Autodesk Fusion 360 part; units mm, degrees
note: some values were not read from the file. Set by a fixed rule: which face or edge a step refers to.
(part 2 of 2)
  spline S256 degree 2 poles (23.5362, -10.063) (23.4772, -9.991) (23.4772, -9.8812) knots 0 0 0 1 1 1
  spline S257 degree 2 poles (23.4772, -9.8812) (23.4772, -9.7366) (23.5808, -9.6541) knots 0 0 0 1 1 1
  spline S258 degree 2 poles (23.5808, -9.6541) (23.7057, -9.5552) (23.9874, -9.5552) knots 0 0 0 1 1 1
  spline S259 degree 2 poles (23.9874, -9.6814) (23.7411, -9.6814) (23.6596, -9.739) knots 0 0 0 1 1 1
  spline S260 degree 2 poles (23.6596, -9.739) (23.5781, -9.7966) (23.5781, -9.8812) knots 0 0 0 1 1 1
  spline S261 degree 2 poles (23.5781, -9.8812) (23.5781, -9.9658) (23.66, -10.0234) knots 0 0 0 1 1 1
  spline S262 degree 2 poles (23.66, -10.0234) (23.7418, -10.0811) (23.9874, -10.0811) knots 0 0 0 1 1 1
  spline S263 degree 2 poles (23.9874, -10.0811) (24.2343, -10.0811) (24.3155, -10.0234) knots 0 0 0 1 1 1
  spline S264 degree 2 poles (24.3155, -10.0234) (24.3967, -9.9658) (24.3967, -9.8799) knots 0 0 0 1 1 1
  spline S265 degree 2 poles (24.3967, -9.8799) (24.3967, -9.7953) (24.325, -9.7448) knots 0 0 0 1 1 1
  spline S266 degree 2 poles (24.325, -9.7448) (24.2336, -9.6814) (23.9874, -9.6814) knots 0 0 0 1 1 1
  line L84 (23.4942, -14.607) -> (23.7336, -14.607)
  line L85 (23.7336, -14.607) -> (23.7336, -14.1732)
  line L86 (23.7336, -14.1732) -> (23.8462, -14.1732)
  line L87 (23.8462, -14.1732) -> (24.4942, -14.6295)
  line L88 (24.4942, -14.6295) -> (24.4942, -14.7298)
  line L89 (24.4942, -14.7298) -> (23.8462, -14.7298)
  line L90 (23.8462, -14.7298) -> (23.8462, -14.8648)
  line L91 (23.8462, -14.8648) -> (23.7336, -14.8648)
  line L92 (23.7336, -14.8648) -> (23.7336, -14.7298)
  line L93 (23.7336, -14.7298) -> (23.4942, -14.7298)
  line L94 (23.4942, -14.7298) -> (23.4942, -14.607)
  line L95 (23.8462, -14.607) -> (24.2971, -14.607)
  line L96 (24.2971, -14.607) -> (23.8462, -14.2939)
  line L97 (23.8462, -14.2939) -> (23.8462, -14.607)
  spline S267 degree 2 poles (23.9874, -14.9904) (24.1647, -14.9904) (24.2729, -15.0269) knots 0 0 0 1 1 1
  spline S268 degree 2 poles (24.2729, -15.0269) (24.381, -15.0633) (24.4396, -15.1353) knots 0 0 0 1 1 1
  spline S269 degree 2 poles (24.4396, -15.1353) (24.4983, -15.2073) (24.4983, -15.3164) knots 0 0 0 1 1 1
  spline S270 degree 2 poles (24.4983, -15.3164) (24.4983, -15.3969) (24.4659, -15.4576) knots 0 0 0 1 1 1
  spline S271 degree 2 poles (24.4659, -15.4576) (24.4335, -15.5183) (24.3724, -15.5579) knots 0 0 0 1 1 1
  spline S272 degree 2 poles (24.3724, -15.5579) (24.3114, -15.5975) (24.2237, -15.62) knots 0 0 0 1 1 1
  spline S273 degree 2 poles (24.2237, -15.62) (24.1361, -15.6425) (23.9874, -15.6425) knots 0 0 0 1 1 1
  spline S274 degree 2 poles (23.9874, -15.6425) (23.8114, -15.6425) (23.7033, -15.6063) knots 0 0 0 1 1 1
  spline S275 degree 2 poles (23.7033, -15.6063) (23.5952, -15.5702) (23.5362, -15.4982) knots 0 0 0 1 1 1
  spline S276 degree 2 poles (23.5362, -15.4982) (23.4772, -15.4262) (23.4772, -15.3164) knots 0 0 0 1 1 1
  spline S277 degree 2 poles (23.4772, -15.3164) (23.4772, -15.1718) (23.5808, -15.0893) knots 0 0 0 1 1 1
  spline S278 degree 2 poles (23.5808, -15.0893) (23.7057, -14.9904) (23.9874, -14.9904) knots 0 0 0 1 1 1
  spline S279 degree 2 poles (23.9874, -15.1166) (23.7411, -15.1166) (23.6596, -15.1742) knots 0 0 0 1 1 1
  spline S280 degree 2 poles (23.6596, -15.1742) (23.5781, -15.2318) (23.5781, -15.3164) knots 0 0 0 1 1 1
  spline S281 degree 2 poles (23.5781, -15.3164) (23.5781, -15.401) (23.66, -15.4586) knots 0 0 0 1 1 1
  spline S282 degree 2 poles (23.66, -15.4586) (23.7418, -15.5163) (23.9874, -15.5163) knots 0 0 0 1 1 1
  spline S283 degree 2 poles (23.9874, -15.5163) (24.2343, -15.5163) (24.3155, -15.4586) knots 0 0 0 1 1 1
  spline S284 degree 2 poles (24.3155, -15.4586) (24.3967, -15.401) (24.3967, -15.3151) knots 0 0 0 1 1 1
  spline S285 degree 2 poles (24.3967, -15.3151) (24.3967, -15.2305) (24.325, -15.18) knots 0 0 0 1 1 1
  spline S286 degree 2 poles (24.325, -15.18) (24.2336, -15.1166) (23.9874, -15.1166) knots 0 0 0 1 1 1
  spline S287 degree 2 poles (23.9874, -15.7673) (24.1647, -15.7673) (24.2729, -15.8038) knots 0 0 0 1 1 1
  spline S288 degree 2 poles (24.2729, -15.8038) (24.381, -15.8403) (24.4396, -15.9123) knots 0 0 0 1 1 1
  spline S289 degree 2 poles (24.4396, -15.9123) (24.4983, -15.9842) (24.4983, -16.0934) knots 0 0 0 1 1 1
  spline S290 degree 2 poles (24.4983, -16.0934) (24.4983, -16.1739) (24.4659, -16.2346) knots 0 0 0 1 1 1
  spline S291 degree 2 poles (24.4659, -16.2346) (24.4335, -16.2953) (24.3724, -16.3348) knots 0 0 0 1 1 1
  spline S292 degree 2 poles (24.3724, -16.3348) (24.3114, -16.3744) (24.2237, -16.3969) knots 0 0 0 1 1 1
  spline S293 degree 2 poles (24.2237, -16.3969) (24.1361, -16.4194) (23.9874, -16.4194) knots 0 0 0 1 1 1
  spline S294 degree 2 poles (23.9874, -16.4194) (23.8114, -16.4194) (23.7033, -16.3833) knots 0 0 0 1 1 1
  spline S295 degree 2 poles (23.7033, -16.3833) (23.5952, -16.3471) (23.5362, -16.2751) knots 0 0 0 1 1 1
  spline S296 degree 2 poles (23.5362, -16.2751) (23.4772, -16.2032) (23.4772, -16.0934) knots 0 0 0 1 1 1
  spline S297 degree 2 poles (23.4772, -16.0934) (23.4772, -15.9487) (23.5808, -15.8662) knots 0 0 0 1 1 1
  spline S298 degree 2 poles (23.5808, -15.8662) (23.7057, -15.7673) (23.9874, -15.7673) knots 0 0 0 1 1 1
  spline S299 degree 2 poles (23.9874, -15.8935) (23.7411, -15.8935) (23.6596, -15.9511) knots 0 0 0 1 1 1
  spline S300 degree 2 poles (23.6596, -15.9511) (23.5781, -16.0088) (23.5781, -16.0934) knots 0 0 0 1 1 1
  spline S301 degree 2 poles (23.5781, -16.0934) (23.5781, -16.1779) (23.66, -16.2356) knots 0 0 0 1 1 1
  spline S302 degree 2 poles (23.66, -16.2356) (23.7418, -16.2932) (23.9874, -16.2932) knots 0 0 0 1 1 1
  spline S303 degree 2 poles (23.9874, -16.2932) (24.2343, -16.2932) (24.3155, -16.2356) knots 0 0 0 1 1 1
  spline S304 degree 2 poles (24.3155, -16.2356) (24.3967, -16.1779) (24.3967, -16.092) knots 0 0 0 1 1 1
  spline S305 degree 2 poles (24.3967, -16.092) (24.3967, -16.0074) (24.325, -15.9569) knots 0 0 0 1 1 1
  spline S306 degree 2 poles (24.325, -15.9569) (24.2336, -15.8935) (23.9874, -15.8935) knots 0 0 0 1 1 1
  line L98 (18.9618, -23.4484) -> (18.9618, -24.4484)
  line L99 (18.9618, -24.4484) -> (18.5184, -24.4484)
  spline S307 degree 2 poles (18.5184, -24.4484) (18.3847, -24.4484) (18.3151, -24.4215) knots 0 0 0 1 1 1
  spline S308 degree 2 poles (18.3151, -24.4215) (18.2455, -24.3945) (18.2039, -24.3263) knots 0 0 0 1 1 1
  spline S309 degree 2 poles (18.2039, -24.3263) (18.1623, -24.2581) (18.1623, -24.1755) knots 0 0 0 1 1 1
  spline S310 degree 2 poles (18.1623, -24.1755) (18.1623, -24.0691) (18.2312, -23.9961) knots 0 0 0 1 1 1
  spline S311 degree 2 poles (18.2312, -23.9961) (18.3001, -23.9232) (18.444, -23.9034) knots 0 0 0 1 1 1
  spline S312 degree 2 poles (18.444, -23.9034) (18.3915, -23.8781) (18.3642, -23.8536) knots 0 0 0 1 1 1
  spline S313 degree 2 poles (18.3642, -23.8536) (18.3062, -23.8004) (18.2544, -23.7206) knots 0 0 0 1 1 1
  line L100 (18.2544, -23.7206) -> (18.0805, -23.4484)
  line L101 (18.0805, -23.4484) -> (18.2469, -23.4484)
  line L102 (18.2469, -23.4484) -> (18.3792, -23.6564)
  spline S314 degree 2 poles (18.3792, -23.6564) (18.4372, -23.7465) (18.4747, -23.7942) knots 0 0 0 1 1 1
  spline S315 degree 2 poles (18.4747, -23.7942) (18.5122, -23.842) (18.5419, -23.8611) knots 0 0 0 1 1 1
  spline S316 degree 2 poles (18.5419, -23.8611) (18.5716, -23.8802) (18.6023, -23.8877) knots 0 0 0 1 1 1
  spline S317 degree 2 poles (18.6023, -23.8877) (18.6248, -23.8925) (18.676, -23.8925) knots 0 0 0 1 1 1
  line L103 (18.676, -23.8925) -> (18.8294, -23.8925)
  line L104 (18.8294, -23.8925) -> (18.8294, -23.4484)
  line L105 (18.8294, -23.4484) -> (18.9618, -23.4484)
  line L106 (18.8294, -24.0071) -> (18.545, -24.0071)
  spline S318 degree 2 poles (18.545, -24.0071) (18.4543, -24.0071) (18.4031, -24.0258) knots 0 0 0 1 1 1
  spline S319 degree 2 poles (18.4031, -24.0258) (18.3519, -24.0446) (18.3253, -24.0858) knots 0 0 0 1 1 1
  spline S320 degree 2 poles (18.3253, -24.0858) (18.2987, -24.1271) (18.2987, -24.1755) knots 0 0 0 1 1 1
  spline S321 degree 2 poles (18.2987, -24.1755) (18.2987, -24.2465) (18.3502, -24.2922) knots 0 0 0 1 1 1
  spline S322 degree 2 poles (18.3502, -24.2922) (18.4017, -24.3379) (18.5129, -24.3379) knots 0 0 0 1 1 1
  line L107 (18.5129, -24.3379) -> (18.8294, -24.3379)
  line L108 (18.8294, -24.3379) -> (18.8294, -24.0071)
  line L109 (17.4747, -23.6817) -> (17.3479, -23.666)
  spline S323 degree 2 poles (17.3479, -23.666) (17.3779, -23.5548) (17.459, -23.4934) knots 0 0 0 1 1 1
  spline S324 degree 2 poles (17.459, -23.4934) (17.5402, -23.432) (17.6664, -23.432) knots 0 0 0 1 1 1
  spline S325 degree 2 poles (17.6664, -23.432) (17.8253, -23.432) (17.9185, -23.5299) knots 0 0 0 1 1 1
  spline S326 degree 2 poles (17.9185, -23.5299) (18.0116, -23.6278) (18.0116, -23.8045) knots 0 0 0 1 1 1
  spline S327 degree 2 poles (18.0116, -23.8045) (18.0116, -23.9873) (17.9174, -24.0882) knots 0 0 0 1 1 1
  spline S328 degree 2 poles (17.9174, -24.0882) (17.8233, -24.1892) (17.6732, -24.1892) knots 0 0 0 1 1 1
  spline S329 degree 2 poles (17.6732, -24.1892) (17.5279, -24.1892) (17.4358, -24.0903) knots 0 0 0 1 1 1
  spline S330 degree 2 poles (17.4358, -24.0903) (17.3438, -23.9914) (17.3438, -23.812) knots 0 0 0 1 1 1
  spline S331 degree 2 poles (17.3438, -23.812) (17.3438, -23.8011) (17.3444, -23.7792) knots 0 0 0 1 1 1
  line L110 (17.3444, -23.7792) -> (17.8847, -23.7792)
  spline S332 degree 2 poles (17.8847, -23.7792) (17.8779, -23.6599) (17.8172, -23.5964) knots 0 0 0 1 1 1
  spline S333 degree 2 poles (17.8172, -23.5964) (17.7564, -23.533) (17.6657, -23.533) knots 0 0 0 1 1 1
  spline S334 degree 2 poles (17.6657, -23.533) (17.5982, -23.533) (17.5504, -23.5685) knots 0 0 0 1 1 1
  spline S335 degree 2 poles (17.5504, -23.5685) (17.5027, -23.6039) (17.4747, -23.6817) knots 0 0 0 1 1 1
  line L111 (17.8779, -23.8802) -> (17.4734, -23.8802)
  spline S336 degree 2 poles (17.4734, -23.8802) (17.4815, -23.9716) (17.5197, -24.0173) knots 0 0 0 1 1 1
  spline S337 degree 2 poles (17.5197, -24.0173) (17.5784, -24.0882) (17.6719, -24.0882) knots 0 0 0 1 1 1
  spline S338 degree 2 poles (17.6719, -24.0882) (17.7564, -24.0882) (17.8141, -24.0316) knots 0 0 0 1 1 1
  spline S339 degree 2 poles (17.8141, -24.0316) (17.8717, -23.975) (17.8779, -23.8802) knots 0 0 0 1 1 1
  line L112 (17.2428, -23.6646) -> (17.1214, -23.6837)
  spline S340 degree 2 poles (17.1214, -23.6837) (17.1112, -23.6107) (17.0644, -23.5719) knots 0 0 0 1 1 1
  spline S341 degree 2 poles (17.0644, -23.5719) (17.0177, -23.533) (16.9338, -23.533) knots 0 0 0 1 1 1
  spline S342 degree 2 poles (16.9338, -23.533) (16.8492, -23.533) (16.8083, -23.5674) knots 0 0 0 1 1 1
  spline S343 degree 2 poles (16.8083, -23.5674) (16.7674, -23.6019) (16.7674, -23.6483) knots 0 0 0 1 1 1
  spline S344 degree 2 poles (16.7674, -23.6483) (16.7674, -23.6899) (16.8035, -23.7137) knots 0 0 0 1 1 1
  spline S345 degree 2 poles (16.8035, -23.7137) (16.8288, -23.7301) (16.929, -23.7554) knots 0 0 0 1 1 1
  spline S346 degree 2 poles (16.929, -23.7554) (17.0641, -23.7895) (17.1163, -23.8144) knots 0 0 0 1 1 1
  spline S347 degree 2 poles (17.1163, -23.8144) (17.1685, -23.8393) (17.1954, -23.8833) knots 0 0 0 1 1 1
  spline S348 degree 2 poles (17.1954, -23.8833) (17.2223, -23.9273) (17.2223, -23.9805) knots 0 0 0 1 1 1
  spline S349 degree 2 poles (17.2223, -23.9805) (17.2223, -24.0289) (17.2002, -24.0702) knots 0 0 0 1 1 1
  spline S350 degree 2 poles (17.2002, -24.0702) (17.178, -24.1114) (17.1398, -24.1387) knots 0 0 0 1 1 1
  spline S351 degree 2 poles (17.1398, -24.1387) (17.1112, -24.1599) (17.0617, -24.1745) knots 0 0 0 1 1 1
  spline S352 degree 2 poles (17.0617, -24.1745) (17.0122, -24.1892) (16.9556, -24.1892) knots 0 0 0 1 1 1
  spline S353 degree 2 poles (16.9556, -24.1892) (16.8704, -24.1892) (16.8059, -24.1646) knots 0 0 0 1 1 1
  spline S354 degree 2 poles (16.8059, -24.1646) (16.7414, -24.1401) (16.7107, -24.0981) knots 0 0 0 1 1 1
  spline S355 degree 2 poles (16.7107, -24.0981) (16.68, -24.0562) (16.6685, -23.9859) knots 0 0 0 1 1 1
  line L113 (16.6685, -23.9859) -> (16.7885, -23.9695)
  spline S356 degree 2 poles (16.7885, -23.9695) (16.7967, -24.0255) (16.8359, -24.0569) knots 0 0 0 1 1 1
  spline S357 degree 2 poles (16.8359, -24.0569) (16.8751, -24.0882) (16.9468, -24.0882) knots 0 0 0 1 1 1
  spline S358 degree 2 poles (16.9468, -24.0882) (17.0313, -24.0882) (17.0675, -24.0603) knots 0 0 0 1 1 1
  spline S359 degree 2 poles (17.0675, -24.0603) (17.1037, -24.0323) (17.1037, -23.9948) knots 0 0 0 1 1 1
  spline S360 degree 2 poles (17.1037, -23.9948) (17.1037, -23.9709) (17.0886, -23.9518) knots 0 0 0 1 1 1
  spline S361 degree 2 poles (17.0886, -23.9518) (17.0736, -23.932) (17.0416, -23.9191) knots 0 0 0 1 1 1
  spline S362 degree 2 poles (17.0416, -23.9191) (17.0232, -23.9122) (16.9331, -23.8877) knots 0 0 0 1 1 1
  spline S363 degree 2 poles (16.9331, -23.8877) (16.8028, -23.8529) (16.7513, -23.8307) knots 0 0 0 1 1 1
  spline S364 degree 2 poles (16.7513, -23.8307) (16.6998, -23.8086) (16.6705, -23.7663) knots 0 0 0 1 1 1
  spline S365 degree 2 poles (16.6705, -23.7663) (16.6412, -23.724) (16.6412, -23.6612) knots 0 0 0 1 1 1
  spline S366 degree 2 poles (16.6412, -23.6612) (16.6412, -23.5998) (16.677, -23.5456) knots 0 0 0 1 1 1
  spline S367 degree 2 poles (16.677, -23.5456) (16.7128, -23.4914) (16.7803, -23.4617) knots 0 0 0 1 1 1
  spline S368 degree 2 poles (16.7803, -23.4617) (16.8479, -23.432) (16.9331, -23.432) knots 0 0 0 1 1 1
  spline S369 degree 2 poles (16.9331, -23.432) (17.0743, -23.432) (17.1483, -23.4907) knots 0 0 0 1 1 1
  spline S370 degree 2 poles (17.1483, -23.4907) (17.2223, -23.5494) (17.2428, -23.6646) knots 0 0 0 1 1 1
  spline S371 degree 2 poles (16.5409, -23.8106) (16.5409, -24.0118) (16.429, -24.1087) knots 0 0 0 1 1 1
  spline S372 degree 2 poles (16.429, -24.1087) (16.3356, -24.1892) (16.2012, -24.1892) knots 0 0 0 1 1 1
  spline S373 degree 2 poles (16.2012, -24.1892) (16.0518, -24.1892) (15.957, -24.0913) knots 0 0 0 1 1 1
  spline S374 degree 2 poles (15.957, -24.0913) (15.8622, -23.9934) (15.8622, -23.8208) knots 0 0 0 1 1 1
  spline S375 degree 2 poles (15.8622, -23.8208) (15.8622, -23.681) (15.9041, -23.6009) knots 0 0 0 1 1 1
  spline S376 degree 2 poles (15.9041, -23.6009) (15.9461, -23.5207) (16.0262, -23.4764) knots 0 0 0 1 1 1
  spline S377 degree 2 poles (16.0262, -23.4764) (16.1064, -23.432) (16.2012, -23.432) knots 0 0 0 1 1 1
  spline S378 degree 2 poles (16.2012, -23.432) (16.3533, -23.432) (16.4471, -23.5296) knots 0 0 0 1 1 1
  spline S379 degree 2 poles (16.4471, -23.5296) (16.5409, -23.6271) (16.5409, -23.8106) knots 0 0 0 1 1 1
  spline S380 degree 2 poles (16.4147, -23.8106) (16.4147, -23.6715) (16.354, -23.6022) knots 0 0 0 1 1 1
  spline S381 degree 2 poles (16.354, -23.6022) (16.2933, -23.533) (16.2012, -23.533) knots 0 0 0 1 1 1
  spline S382 degree 2 poles (16.2012, -23.533) (16.1098, -23.533) (16.0491, -23.6026) knots 0 0 0 1 1 1
  spline S383 degree 2 poles (16.0491, -23.6026) (15.9884, -23.6721) (15.9884, -23.8147) knots 0 0 0 1 1 1
  spline S384 degree 2 poles (15.9884, -23.8147) (15.9884, -23.9491) (16.0494, -24.0183) knots 0 0 0 1 1 1
  spline S385 degree 2 poles (16.0494, -24.0183) (16.1105, -24.0876) (16.2012, -24.0876) knots 0 0 0 1 1 1
  spline S386 degree 2 poles (16.2012, -24.0876) (16.2933, -24.0876) (16.354, -24.0187) knots 0 0 0 1 1 1
  spline S387 degree 2 poles (16.354, -24.0187) (16.4147, -23.9498) (16.4147, -23.8106) knots 0 0 0 1 1 1
  line L114 (15.721, -23.4484) -> (15.721, -24.4484)
  line L115 (15.721, -24.4484) -> (15.5982, -24.4484)
  line L116 (15.5982, -24.4484) -> (15.5982, -23.4484)
  line L117 (15.5982, -23.4484) -> (15.721, -23.4484)
  line L118 (14.9331, -23.4484) -> (14.9331, -23.5548)
  spline S388 degree 2 poles (14.9331, -23.5548) (15.0177, -23.432) (15.163, -23.432) knots 0 0 0 1 1 1
  spline S389 degree 2 poles (15.163, -23.432) (15.2271, -23.432) (15.2827, -23.4566) knots 0 0 0 1 1 1
  spline S390 degree 2 poles (15.2827, -23.4566) (15.3383, -23.4811) (15.3652, -23.5183) knots 0 0 0 1 1 1
  spline S391 degree 2 poles (15.3652, -23.5183) (15.3922, -23.5555) (15.4031, -23.6094) knots 0 0 0 1 1 1
  spline S392 degree 2 poles (15.4031, -23.6094) (15.4106, -23.6455) (15.4106, -23.724) knots 0 0 0 1 1 1
  line L119 (15.4106, -23.724) -> (15.4106, -24.1728)
  line L120 (15.4106, -24.1728) -> (15.2878, -24.1728)
  line L121 (15.2878, -24.1728) -> (15.2878, -23.771)
  spline S393 degree 2 poles (15.2878, -23.771) (15.2878, -23.6749) (15.2803, -23.6414) knots 0 0 0 1 1 1
  spline S394 degree 2 poles (15.2803, -23.6414) (15.2687, -23.593) (15.2312, -23.5654) knots 0 0 0 1 1 1
  spline S395 degree 2 poles (15.2312, -23.5654) (15.1937, -23.5378) (15.1384, -23.5378) knots 0 0 0 1 1 1
  spline S396 degree 2 poles (15.1384, -23.5378) (15.0832, -23.5378) (15.0348, -23.5661) knots 0 0 0 1 1 1
  spline S397 degree 2 poles (15.0348, -23.5661) (14.9863, -23.5944) (14.9662, -23.6431) knots 0 0 0 1 1 1
  spline S398 degree 2 poles (14.9662, -23.6431) (14.9461, -23.6919) (14.9461, -23.7847) knots 0 0 0 1 1 1
  line L122 (14.9461, -23.7847) -> (14.9461, -24.1728)
  line L123 (14.9461, -24.1728) -> (14.8233, -24.1728)
  line L124 (14.8233, -24.1728) -> (14.8233, -23.4484)
  line L125 (14.8233, -23.4484) -> (14.9331, -23.4484)
  line L126 (14.3629, -23.5582) -> (14.3451, -23.4498)
  spline S399 degree 2 poles (14.3451, -23.4498) (14.397, -23.4388) (14.4379, -23.4388) knots 0 0 0 1 1 1
  spline S400 degree 2 poles (14.4379, -23.4388) (14.5047, -23.4388) (14.5416, -23.46) knots 0 0 0 1 1 1
  spline S401 degree 2 poles (14.5416, -23.46) (14.5784, -23.4811) (14.5934, -23.5156) knots 0 0 0 1 1 1
  spline S402 degree 2 poles (14.5934, -23.5156) (14.6084, -23.55) (14.6084, -23.6605) knots 0 0 0 1 1 1
  line L127 (14.6084, -23.6605) -> (14.6084, -24.0773)
  line L128 (14.6084, -24.0773) -> (14.6985, -24.0773)
  line L129 (14.6985, -24.0773) -> (14.6985, -24.1728)
  line L130 (14.6985, -24.1728) -> (14.6084, -24.1728)
  line L131 (14.6084, -24.1728) -> (14.6084, -24.3522)
  line L132 (14.6084, -24.3522) -> (14.4863, -24.4259)
  line L133 (14.4863, -24.4259) -> (14.4863, -24.1728)
  line L134 (14.4863, -24.1728) -> (14.3629, -24.1728)
  line L135 (14.3629, -24.1728) -> (14.3629, -24.0773)
  line L136 (14.3629, -24.0773) -> (14.4863, -24.0773)
  line L137 (14.4863, -24.0773) -> (14.4863, -23.6537)
  spline S403 degree 2 poles (14.4863, -23.6537) (14.4863, -23.6012) (14.4798, -23.5862) knots 0 0 0 1 1 1
  spline S404 degree 2 poles (14.4798, -23.5862) (14.4734, -23.5712) (14.4587, -23.5623) knots 0 0 0 1 1 1
  spline S405 degree 2 poles (14.4587, -23.5623) (14.444, -23.5534) (14.4167, -23.5534) knots 0 0 0 1 1 1
  spline S406 degree 2 poles (14.4167, -23.5534) (14.3963, -23.5534) (14.3629, -23.5582) knots 0 0 0 1 1 1
  line L138 (14.2421, -24.3072) -> (14.2421, -24.4484)
  line L139 (14.2421, -24.4484) -> (14.1193, -24.4484)
  line L140 (14.1193, -24.4484) -> (14.1193, -24.3072)
  line L141 (14.1193, -24.3072) -> (14.2421, -24.3072)
  line L142 (14.2421, -23.4484) -> (14.2421, -24.1728)
  line L143 (14.2421, -24.1728) -> (14.1193, -24.1728)
  line L144 (14.1193, -24.1728) -> (14.1193, -23.4484)
  line L145 (14.1193, -23.4484) -> (14.2421, -23.4484)
  spline S407 degree 2 poles (13.9781, -23.8106) (13.9781, -24.0118) (13.8663, -24.1087) knots 0 0 0 1 1 1
  spline S408 degree 2 poles (13.8663, -24.1087) (13.7728, -24.1892) (13.6384, -24.1892) knots 0 0 0 1 1 1
  spline S409 degree 2 poles (13.6384, -24.1892) (13.4891, -24.1892) (13.3942, -24.0913) knots 0 0 0 1 1 1
  spline S410 degree 2 poles (13.3942, -24.0913) (13.2994, -23.9934) (13.2994, -23.8208) knots 0 0 0 1 1 1
  spline S411 degree 2 poles (13.2994, -23.8208) (13.2994, -23.681) (13.3414, -23.6009) knots 0 0 0 1 1 1
  spline S412 degree 2 poles (13.3414, -23.6009) (13.3833, -23.5207) (13.4635, -23.4764) knots 0 0 0 1 1 1
  spline S413 degree 2 poles (13.4635, -23.4764) (13.5436, -23.432) (13.6384, -23.432) knots 0 0 0 1 1 1
  spline S414 degree 2 poles (13.6384, -23.432) (13.7906, -23.432) (13.8843, -23.5296) knots 0 0 0 1 1 1
  spline S415 degree 2 poles (13.8843, -23.5296) (13.9781, -23.6271) (13.9781, -23.8106) knots 0 0 0 1 1 1
  spline S416 degree 2 poles (13.8519, -23.8106) (13.8519, -23.6715) (13.7912, -23.6022) knots 0 0 0 1 1 1
  spline S417 degree 2 poles (13.7912, -23.6022) (13.7305, -23.533) (13.6384, -23.533) knots 0 0 0 1 1 1
  spline S418 degree 2 poles (13.6384, -23.533) (13.547, -23.533) (13.4863, -23.6026) knots 0 0 0 1 1 1
  spline S419 degree 2 poles (13.4863, -23.6026) (13.4256, -23.6721) (13.4256, -23.8147) knots 0 0 0 1 1 1
  spline S420 degree 2 poles (13.4256, -23.8147) (13.4256, -23.9491) (13.4867, -24.0183) knots 0 0 0 1 1 1
  spline S421 degree 2 poles (13.4867, -24.0183) (13.5477, -24.0876) (13.6384, -24.0876) knots 0 0 0 1 1 1
  spline S422 degree 2 poles (13.6384, -24.0876) (13.7305, -24.0876) (13.7912, -24.0187) knots 0 0 0 1 1 1
  spline S423 degree 2 poles (13.7912, -24.0187) (13.8519, -23.9498) (13.8519, -23.8106) knots 0 0 0 1 1 1
  line L146 (13.1555, -23.4484) -> (13.1555, -24.1728)
  line L147 (13.1555, -24.1728) -> (13.045, -24.1728)
  line L148 (13.045, -24.1728) -> (13.045, -24.0698)
  spline S424 degree 2 poles (13.045, -24.0698) (12.9652, -24.1892) (12.8144, -24.1892) knots 0 0 0 1 1 1
  spline S425 degree 2 poles (12.8144, -24.1892) (12.7489, -24.1892) (12.694, -24.1657) knots 0 0 0 1 1 1
  spline S426 degree 2 poles (12.694, -24.1657) (12.6391, -24.1421) (12.6118, -24.1039) knots 0 0 0 1 1 1
  spline S427 degree 2 poles (12.6118, -24.1039) (12.5846, -24.0657) (12.5736, -24.0132) knots 0 0 0 1 1 1
  spline S428 degree 2 poles (12.5736, -24.0132) (12.5668, -23.9791) (12.5668, -23.8938) knots 0 0 0 1 1 1
  line L149 (12.5668, -23.8938) -> (12.5668, -23.4484)
  line L150 (12.5668, -23.4484) -> (12.6896, -23.4484)
  line L151 (12.6896, -23.4484) -> (12.6896, -23.8891)
  spline S429 degree 2 poles (12.6896, -23.8891) (12.6896, -23.9641) (12.7039, -24.0013) knots 0 0 0 1 1 1
  spline S430 degree 2 poles (12.7039, -24.0013) (12.7182, -24.0384) (12.7547, -24.0606) knots 0 0 0 1 1 1
  spline S431 degree 2 poles (12.7547, -24.0606) (12.7912, -24.0828) (12.8403, -24.0828) knots 0 0 0 1 1 1
  spline S432 degree 2 poles (12.8403, -24.0828) (12.9188, -24.0828) (12.9758, -24.033) knots 0 0 0 1 1 1
  spline S433 degree 2 poles (12.9758, -24.033) (13.0327, -23.9832) (13.0327, -23.844) knots 0 0 0 1 1 1
  line L152 (13.0327, -23.844) -> (13.0327, -23.4484)
  line L153 (13.0327, -23.4484) -> (13.1555, -23.4484)
  line L154 (11.7223, -23.5582) -> (11.7046, -23.4498)
  spline S434 degree 2 poles (11.7046, -23.4498) (11.7564, -23.4388) (11.7974, -23.4388) knots 0 0 0 1 1 1
  spline S435 degree 2 poles (11.7974, -23.4388) (11.8642, -23.4388) (11.9011, -23.46) knots 0 0 0 1 1 1
  spline S436 degree 2 poles (11.9011, -23.46) (11.9379, -23.4811) (11.9529, -23.5156) knots 0 0 0 1 1 1
  spline S437 degree 2 poles (11.9529, -23.5156) (11.9679, -23.55) (11.9679, -23.6605) knots 0 0 0 1 1 1
  line L155 (11.9679, -23.6605) -> (11.9679, -24.0773)
  line L156 (11.9679, -24.0773) -> (12.0579, -24.0773)
  line L157 (12.0579, -24.0773) -> (12.0579, -24.1728)
  line L158 (12.0579, -24.1728) -> (11.9679, -24.1728)
  line L159 (11.9679, -24.1728) -> (11.9679, -24.3522)
  line L160 (11.9679, -24.3522) -> (11.8458, -24.4259)
  line L161 (11.8458, -24.4259) -> (11.8458, -24.1728)
  line L162 (11.8458, -24.1728) -> (11.7223, -24.1728)
  line L163 (11.7223, -24.1728) -> (11.7223, -24.0773)
  line L164 (11.7223, -24.0773) -> (11.8458, -24.0773)
  line L165 (11.8458, -24.0773) -> (11.8458, -23.6537)
  spline S438 degree 2 poles (11.8458, -23.6537) (11.8458, -23.6012) (11.8393, -23.5862) knots 0 0 0 1 1 1
  spline S439 degree 2 poles (11.8393, -23.5862) (11.8328, -23.5712) (11.8182, -23.5623) knots 0 0 0 1 1 1
  spline S440 degree 2 poles (11.8182, -23.5623) (11.8035, -23.5534) (11.7762, -23.5534) knots 0 0 0 1 1 1
  spline S441 degree 2 poles (11.7762, -23.5534) (11.7558, -23.5534) (11.7223, -23.5582) knots 0 0 0 1 1 1
  line L166 (11.1064, -23.6817) -> (10.9795, -23.666)
  spline S442 degree 2 poles (10.9795, -23.666) (11.0095, -23.5548) (11.0907, -23.4934) knots 0 0 0 1 1 1
  spline S443 degree 2 poles (11.0907, -23.4934) (11.1719, -23.432) (11.2981, -23.432) knots 0 0 0 1 1 1
  spline S444 degree 2 poles (11.2981, -23.432) (11.457, -23.432) (11.5501, -23.5299) knots 0 0 0 1 1 1
  spline S445 degree 2 poles (11.5501, -23.5299) (11.6432, -23.6278) (11.6432, -23.8045) knots 0 0 0 1 1 1
  spline S446 degree 2 poles (11.6432, -23.8045) (11.6432, -23.9873) (11.5491, -24.0882) knots 0 0 0 1 1 1
  spline S447 degree 2 poles (11.5491, -24.0882) (11.4549, -24.1892) (11.3049, -24.1892) knots 0 0 0 1 1 1
  spline S448 degree 2 poles (11.3049, -24.1892) (11.1596, -24.1892) (11.0675, -24.0903) knots 0 0 0 1 1 1
  spline S449 degree 2 poles (11.0675, -24.0903) (10.9754, -23.9914) (10.9754, -23.812) knots 0 0 0 1 1 1
  spline S450 degree 2 poles (10.9754, -23.812) (10.9754, -23.8011) (10.9761, -23.7792) knots 0 0 0 1 1 1
  line L167 (10.9761, -23.7792) -> (11.5163, -23.7792)
  spline S451 degree 2 poles (11.5163, -23.7792) (11.5095, -23.6599) (11.4488, -23.5964) knots 0 0 0 1 1 1
  spline S452 degree 2 poles (11.4488, -23.5964) (11.3881, -23.533) (11.2974, -23.533) knots 0 0 0 1 1 1
  spline S453 degree 2 poles (11.2974, -23.533) (11.2298, -23.533) (11.1821, -23.5685) knots 0 0 0 1 1 1
  spline S454 degree 2 poles (11.1821, -23.5685) (11.1343, -23.6039) (11.1064, -23.6817) knots 0 0 0 1 1 1
  line L168 (11.5095, -23.8802) -> (11.105, -23.8802)
  spline S455 degree 2 poles (11.105, -23.8802) (11.1132, -23.9716) (11.1514, -24.0173) knots 0 0 0 1 1 1
  spline S456 degree 2 poles (11.1514, -24.0173) (11.2101, -24.0882) (11.3035, -24.0882) knots 0 0 0 1 1 1
  spline S457 degree 2 poles (11.3035, -24.0882) (11.3881, -24.0882) (11.4457, -24.0316) knots 0 0 0 1 1 1
  spline S458 degree 2 poles (11.4457, -24.0316) (11.5034, -23.975) (11.5095, -23.8802) knots 0 0 0 1 1 1
  line L169 (10.8745, -23.6646) -> (10.753, -23.6837)
  spline S459 degree 2 poles (10.753, -23.6837) (10.7428, -23.6107) (10.6961, -23.5719) knots 0 0 0 1 1 1
  spline S460 degree 2 poles (10.6961, -23.5719) (10.6494, -23.533) (10.5655, -23.533) knots 0 0 0 1 1 1
  spline S461 degree 2 poles (10.5655, -23.533) (10.4809, -23.533) (10.4399, -23.5674) knots 0 0 0 1 1 1
  spline S462 degree 2 poles (10.4399, -23.5674) (10.399, -23.6019) (10.399, -23.6483) knots 0 0 0 1 1 1
  spline S463 degree 2 poles (10.399, -23.6483) (10.399, -23.6899) (10.4352, -23.7137) knots 0 0 0 1 1 1
  spline S464 degree 2 poles (10.4352, -23.7137) (10.4604, -23.7301) (10.5607, -23.7554) knots 0 0 0 1 1 1
  spline S465 degree 2 poles (10.5607, -23.7554) (10.6957, -23.7895) (10.7479, -23.8144) knots 0 0 0 1 1 1
  spline S466 degree 2 poles (10.7479, -23.8144) (10.8001, -23.8393) (10.827, -23.8833) knots 0 0 0 1 1 1
  spline S467 degree 2 poles (10.827, -23.8833) (10.854, -23.9273) (10.854, -23.9805) knots 0 0 0 1 1 1
  spline S468 degree 2 poles (10.854, -23.9805) (10.854, -24.0289) (10.8318, -24.0702) knots 0 0 0 1 1 1
  spline S469 degree 2 poles (10.8318, -24.0702) (10.8097, -24.1114) (10.7715, -24.1387) knots 0 0 0 1 1 1
  spline S470 degree 2 poles (10.7715, -24.1387) (10.7428, -24.1599) (10.6933, -24.1745) knots 0 0 0 1 1 1
  spline S471 degree 2 poles (10.6933, -24.1745) (10.6439, -24.1892) (10.5873, -24.1892) knots 0 0 0 1 1 1
  spline S472 degree 2 poles (10.5873, -24.1892) (10.502, -24.1892) (10.4376, -24.1646) knots 0 0 0 1 1 1
  spline S473 degree 2 poles (10.4376, -24.1646) (10.3731, -24.1401) (10.3424, -24.0981) knots 0 0 0 1 1 1
  spline S474 degree 2 poles (10.3424, -24.0981) (10.3117, -24.0562) (10.3001, -23.9859) knots 0 0 0 1 1 1
  line L170 (10.3001, -23.9859) -> (10.4202, -23.9695)
  spline S475 degree 2 poles (10.4202, -23.9695) (10.4283, -24.0255) (10.4676, -24.0569) knots 0 0 0 1 1 1
  spline S476 degree 2 poles (10.4676, -24.0569) (10.5068, -24.0882) (10.5784, -24.0882) knots 0 0 0 1 1 1
  spline S477 degree 2 poles (10.5784, -24.0882) (10.663, -24.0882) (10.6991, -24.0603) knots 0 0 0 1 1 1
  spline S478 degree 2 poles (10.6991, -24.0603) (10.7353, -24.0323) (10.7353, -23.9948) knots 0 0 0 1 1 1
  spline S479 degree 2 poles (10.7353, -23.9948) (10.7353, -23.9709) (10.7203, -23.9518) knots 0 0 0 1 1 1
  spline S480 degree 2 poles (10.7203, -23.9518) (10.7053, -23.932) (10.6732, -23.9191) knots 0 0 0 1 1 1
  spline S481 degree 2 poles (10.6732, -23.9191) (10.6548, -23.9122) (10.5648, -23.8877) knots 0 0 0 1 1 1
  spline S482 degree 2 poles (10.5648, -23.8877) (10.4345, -23.8529) (10.383, -23.8307) knots 0 0 0 1 1 1
  spline S483 degree 2 poles (10.383, -23.8307) (10.3315, -23.8086) (10.3021, -23.7663) knots 0 0 0 1 1 1
  spline S484 degree 2 poles (10.3021, -23.7663) (10.2728, -23.724) (10.2728, -23.6612) knots 0 0 0 1 1 1
  spline S485 degree 2 poles (10.2728, -23.6612) (10.2728, -23.5998) (10.3086, -23.5456) knots 0 0 0 1 1 1
  spline S486 degree 2 poles (10.3086, -23.5456) (10.3444, -23.4914) (10.412, -23.4617) knots 0 0 0 1 1 1
  spline S487 degree 2 poles (10.412, -23.4617) (10.4795, -23.432) (10.5648, -23.432) knots 0 0 0 1 1 1
  spline S488 degree 2 poles (10.5648, -23.432) (10.706, -23.432) (10.78, -23.4907) knots 0 0 0 1 1 1
  spline S489 degree 2 poles (10.78, -23.4907) (10.854, -23.5494) (10.8745, -23.6646) knots 0 0 0 1 1 1
  line L171 (9.8588, -23.5582) -> (9.841, -23.4498)
  spline S490 degree 2 poles (9.841, -23.4498) (9.8929, -23.4388) (9.9338, -23.4388) knots 0 0 0 1 1 1
  spline S491 degree 2 poles (9.9338, -23.4388) (10.0006, -23.4388) (10.0375, -23.46) knots 0 0 0 1 1 1
  spline S492 degree 2 poles (10.0375, -23.46) (10.0743, -23.4811) (10.0893, -23.5156) knots 0 0 0 1 1 1
  spline S493 degree 2 poles (10.0893, -23.5156) (10.1043, -23.55) (10.1043, -23.6605) knots 0 0 0 1 1 1
  line L172 (10.1043, -23.6605) -> (10.1043, -24.0773)
  line L173 (10.1043, -24.0773) -> (10.1944, -24.0773)
  line L174 (10.1944, -24.0773) -> (10.1944, -24.1728)
  line L175 (10.1944, -24.1728) -> (10.1043, -24.1728)
  line L176 (10.1043, -24.1728) -> (10.1043, -24.3522)
  line L177 (10.1043, -24.3522) -> (9.9822, -24.4259)
  line L178 (9.9822, -24.4259) -> (9.9822, -24.1728)
  line L179 (9.9822, -24.1728) -> (9.8588, -24.1728)
  line L180 (9.8588, -24.1728) -> (9.8588, -24.0773)
  line L181 (9.8588, -24.0773) -> (9.9822, -24.0773)
  line L182 (9.9822, -24.0773) -> (9.9822, -23.6537)
  spline S494 degree 2 poles (9.9822, -23.6537) (9.9822, -23.6012) (9.9758, -23.5862) knots 0 0 0 1 1 1
  spline S495 degree 2 poles (9.9758, -23.5862) (9.9693, -23.5712) (9.9546, -23.5623) knots 0 0 0 1 1 1
  spline S496 degree 2 poles (9.9546, -23.5623) (9.9399, -23.5534) (9.9127, -23.5534) knots 0 0 0 1 1 1
  spline S497 degree 2 poles (9.9127, -23.5534) (9.8922, -23.5534) (9.8588, -23.5582) knots 0 0 0 1 1 1
  spline S498 degree 2 poles (9.3847, -23.9416) (9.3847, -24.1189) (9.3482, -24.227) knots 0 0 0 1 1 1
  spline S499 degree 2 poles (9.3482, -24.227) (9.3117, -24.3352) (9.2397, -24.3938) knots 0 0 0 1 1 1
  spline S500 degree 2 poles (9.2397, -24.3938) (9.1678, -24.4525) (9.0586, -24.4525) knots 0 0 0 1 1 1
  spline S501 degree 2 poles (9.0586, -24.4525) (8.9781, -24.4525) (8.9174, -24.4201) knots 0 0 0 1 1 1
  spline S502 degree 2 poles (8.9174, -24.4201) (8.8567, -24.3877) (8.8172, -24.3266) knots 0 0 0 1 1 1
  spline S503 degree 2 poles (8.8172, -24.3266) (8.7776, -24.2656) (8.7551, -24.1779) knots 0 0 0 1 1 1
  spline S504 degree 2 poles (8.7551, -24.1779) (8.7326, -24.0903) (8.7326, -23.9416) knots 0 0 0 1 1 1
  spline S505 degree 2 poles (8.7326, -23.9416) (8.7326, -23.7656) (8.7687, -23.6575) knots 0 0 0 1 1 1
  spline S506 degree 2 poles (8.7687, -23.6575) (8.8049, -23.5494) (8.8768, -23.4903) knots 0 0 0 1 1 1
  spline S507 degree 2 poles (8.8768, -23.4903) (8.9488, -23.4313) (9.0586, -23.4313) knots 0 0 0 1 1 1
  spline S508 degree 2 poles (9.0586, -23.4313) (9.2032, -23.4313) (9.2858, -23.535) knots 0 0 0 1 1 1
  spline S509 degree 2 poles (9.2858, -23.535) (9.3847, -23.6599) (9.3847, -23.9416) knots 0 0 0 1 1 1
  spline S510 degree 2 poles (9.2585, -23.9416) (9.2585, -23.6953) (9.2009, -23.6138) knots 0 0 0 1 1 1
  spline S511 degree 2 poles (9.2009, -23.6138) (9.1432, -23.5323) (9.0586, -23.5323) knots 0 0 0 1 1 1
  spline S512 degree 2 poles (9.0586, -23.5323) (8.974, -23.5323) (8.9164, -23.6142) knots 0 0 0 1 1 1
  spline S513 degree 2 poles (8.9164, -23.6142) (8.8588, -23.696) (8.8588, -23.9416) knots 0 0 0 1 1 1
  spline S514 degree 2 poles (8.8588, -23.9416) (8.8588, -24.1885) (8.9164, -24.2697) knots 0 0 0 1 1 1
  spline S515 degree 2 poles (8.9164, -24.2697) (8.974, -24.3509) (9.06, -24.3509) knots 0 0 0 1 1 1
  spline S516 degree 2 poles (9.06, -24.3509) (9.1446, -24.3509) (9.1951, -24.2792) knots 0 0 0 1 1 1
  spline S517 degree 2 poles (9.1951, -24.2792) (9.2585, -24.1878) (9.2585, -23.9416) knots 0 0 0 1 1 1
  line L183 (7.7155, -23.4484) -> (7.7155, -23.5398)
  spline S518 degree 2 poles (7.7155, -23.5398) (7.7844, -23.432) (7.9181, -23.432) knots 0 0 0 1 1 1
  spline S519 degree 2 poles (7.9181, -23.432) (8.0047, -23.432) (8.0774, -23.4798) knots 0 0 0 1 1 1
  spline S520 degree 2 poles (8.0774, -23.4798) (8.15, -23.5275) (8.1899, -23.6131) knots 0 0 0 1 1 1
  spline S521 degree 2 poles (8.1899, -23.6131) (8.2298, -23.6987) (8.2298, -23.8099) knots 0 0 0 1 1 1
  spline S522 degree 2 poles (8.2298, -23.8099) (8.2298, -23.9184) (8.1937, -24.0067) knots 0 0 0 1 1 1
  spline S523 degree 2 poles (8.1937, -24.0067) (8.1575, -24.0951) (8.0852, -24.1421) knots 0 0 0 1 1 1
  spline S524 degree 2 poles (8.0852, -24.1421) (8.0129, -24.1892) (7.9236, -24.1892) knots 0 0 0 1 1 1
  spline S525 degree 2 poles (7.9236, -24.1892) (7.8581, -24.1892) (7.8069, -24.1616) knots 0 0 0 1 1 1
  spline S526 degree 2 poles (7.8069, -24.1616) (7.7558, -24.1339) (7.7237, -24.0896) knots 0 0 0 1 1 1
  line L184 (7.7237, -24.0896) -> (7.7237, -24.4484)
  line L185 (7.7237, -24.4484) -> (7.6016, -24.4484)
  line L186 (7.6016, -24.4484) -> (7.6016, -23.4484)
  line L187 (7.6016, -23.4484) -> (7.7155, -23.4484)
  spline S527 degree 2 poles (8.1036, -23.8099) (8.1036, -23.6708) (8.045, -23.6019) knots 0 0 0 1 1 1
  spline S528 degree 2 poles (8.045, -23.6019) (7.9863, -23.533) (7.9065, -23.533) knots 0 0 0 1 1 1
  spline S529 degree 2 poles (7.9065, -23.533) (7.826, -23.533) (7.7697, -23.5988) knots 0 0 0 1 1 1
  spline S530 degree 2 poles (7.7697, -23.5988) (7.7135, -23.6646) (7.7135, -23.7997) knots 0 0 0 1 1 1
  spline S531 degree 2 poles (7.7135, -23.7997) (7.7135, -23.9484) (7.7708, -24.018) knots 0 0 0 1 1 1
  spline S532 degree 2 poles (7.7708, -24.018) (7.8281, -24.0876) (7.912, -24.0876) knots 0 0 0 1 1 1
  spline S533 degree 2 poles (7.912, -24.0876) (7.9938, -24.0876) (8.0487, -24.0207) knots 0 0 0 1 1 1
  spline S534 degree 2 poles (8.0487, -24.0207) (8.1036, -23.9539) (8.1036, -23.8099) knots 0 0 0 1 1 1
  line L188 (6.9127, -23.6817) -> (6.7858, -23.666)
  spline S535 degree 2 poles (6.7858, -23.666) (6.8158, -23.5548) (6.897, -23.4934) knots 0 0 0 1 1 1
  spline S536 degree 2 poles (6.897, -23.4934) (6.9781, -23.432) (7.1043, -23.432) knots 0 0 0 1 1 1
  spline S537 degree 2 poles (7.1043, -23.432) (7.2633, -23.432) (7.3564, -23.5299) knots 0 0 0 1 1 1
  spline S538 degree 2 poles (7.3564, -23.5299) (7.4495, -23.6278) (7.4495, -23.8045) knots 0 0 0 1 1 1
  spline S539 degree 2 poles (7.4495, -23.8045) (7.4495, -23.9873) (7.3554, -24.0882) knots 0 0 0 1 1 1
  spline S540 degree 2 poles (7.3554, -24.0882) (7.2612, -24.1892) (7.1112, -24.1892) knots 0 0 0 1 1 1
  spline S541 degree 2 poles (7.1112, -24.1892) (6.9659, -24.1892) (6.8738, -24.0903) knots 0 0 0 1 1 1
  spline S542 degree 2 poles (6.8738, -24.0903) (6.7817, -23.9914) (6.7817, -23.812) knots 0 0 0 1 1 1
  spline S543 degree 2 poles (6.7817, -23.812) (6.7817, -23.8011) (6.7824, -23.7792) knots 0 0 0 1 1 1
  line L189 (6.7824, -23.7792) -> (7.3226, -23.7792)
  spline S544 degree 2 poles (7.3226, -23.7792) (7.3158, -23.6599) (7.2551, -23.5964) knots 0 0 0 1 1 1
  spline S545 degree 2 poles (7.2551, -23.5964) (7.1944, -23.533) (7.1036, -23.533) knots 0 0 0 1 1 1
  spline S546 degree 2 poles (7.1036, -23.533) (7.0361, -23.533) (6.9884, -23.5685) knots 0 0 0 1 1 1
  spline S547 degree 2 poles (6.9884, -23.5685) (6.9406, -23.6039) (6.9127, -23.6817) knots 0 0 0 1 1 1
  line L190 (7.3158, -23.8802) -> (6.9113, -23.8802)
  spline S548 degree 2 poles (6.9113, -23.8802) (6.9195, -23.9716) (6.9577, -24.0173) knots 0 0 0 1 1 1
  spline S549 degree 2 poles (6.9577, -24.0173) (7.0163, -24.0882) (7.1098, -24.0882) knots 0 0 0 1 1 1
  spline S550 degree 2 poles (7.1098, -24.0882) (7.1944, -24.0882) (7.252, -24.0316) knots 0 0 0 1 1 1
  spline S551 degree 2 poles (7.252, -24.0316) (7.3097, -23.975) (7.3158, -23.8802) knots 0 0 0 1 1 1
  line L191 (6.6541, -23.3884) -> (6.5348, -23.3706)
  spline S552 degree 2 poles (6.5348, -23.3706) (6.5273, -23.3154) (6.4931, -23.2901) knots 0 0 0 1 1 1
  spline S553 degree 2 poles (6.4931, -23.2901) (6.4474, -23.256) (6.3683, -23.256) knots 0 0 0 1 1 1
  spline S554 degree 2 poles (6.3683, -23.256) (6.283, -23.256) (6.2367, -23.2901) knots 0 0 0 1 1 1
  spline S555 degree 2 poles (6.2367, -23.2901) (6.1903, -23.3243) (6.1739, -23.3856) knots 0 0 0 1 1 1
  spline S556 degree 2 poles (6.1739, -23.3856) (6.1644, -23.4232) (6.165, -23.5432) knots 0 0 0 1 1 1
  spline S557 degree 2 poles (6.165, -23.5432) (6.2455, -23.4484) (6.3656, -23.4484) knots 0 0 0 1 1 1
  spline S558 degree 2 poles (6.3656, -23.4484) (6.515, -23.4484) (6.5968, -23.5562) knots 0 0 0 1 1 1
  spline S559 degree 2 poles (6.5968, -23.5562) (6.6787, -23.664) (6.6787, -23.8147) knots 0 0 0 1 1 1
  spline S560 degree 2 poles (6.6787, -23.8147) (6.6787, -23.9184) (6.6412, -24.006) knots 0 0 0 1 1 1
  spline S561 degree 2 poles (6.6412, -24.006) (6.6037, -24.0937) (6.5324, -24.1414) knots 0 0 0 1 1 1
  spline S562 degree 2 poles (6.5324, -24.1414) (6.4611, -24.1892) (6.3649, -24.1892) knots 0 0 0 1 1 1
  spline S563 degree 2 poles (6.3649, -24.1892) (6.2367, -24.1892) (6.1534, -24.0855) knots 0 0 0 1 1 1
  line L192 (6.1534, -24.0855) -> (6.1534, -24.1728)
  line L193 (6.1534, -24.1728) -> (6.0402, -24.1728)
  line L194 (6.0402, -24.1728) -> (6.0402, -23.5466)
  spline S564 degree 2 poles (6.0402, -23.5466) (6.0402, -23.3775) (6.0747, -23.3069) knots 0 0 0 1 1 1
  spline S565 degree 2 poles (6.0747, -23.3069) (6.1091, -23.2363) (6.1838, -23.1953) knots 0 0 0 1 1 1
  spline S566 degree 2 poles (6.1838, -23.1953) (6.2585, -23.1544) (6.3676, -23.1544) knots 0 0 0 1 1 1
  spline S567 degree 2 poles (6.3676, -23.1544) (6.4972, -23.1544) (6.577, -23.2127) knots 0 0 0 1 1 1
  spline S568 degree 2 poles (6.577, -23.2127) (6.6569, -23.271) (6.6541, -23.3884) knots 0 0 0 1 1 1
  spline S569 degree 2 poles (6.5525, -23.8236) (6.5525, -23.681) (6.4959, -23.6155) knots 0 0 0 1 1 1
  spline S570 degree 2 poles (6.4959, -23.6155) (6.4393, -23.55) (6.354, -23.55) knots 0 0 0 1 1 1
  spline S571 degree 2 poles (6.354, -23.55) (6.2694, -23.55) (6.2121, -23.6152) knots 0 0 0 1 1 1
  spline S572 degree 2 poles (6.2121, -23.6152) (6.1548, -23.6803) (6.1548, -23.8195) knots 0 0 0 1 1 1
  spline S573 degree 2 poles (6.1548, -23.8195) (6.1548, -23.9525) (6.2138, -24.02) knots 0 0 0 1 1 1
  spline S574 degree 2 poles (6.2138, -24.02) (6.2728, -24.0876) (6.356, -24.0876) knots 0 0 0 1 1 1
  spline S575 degree 2 poles (6.356, -24.0876) (6.4379, -24.0876) (6.4952, -24.021) knots 0 0 0 1 1 1
  spline S576 degree 2 poles (6.4952, -24.021) (6.5525, -23.9545) (6.5525, -23.8236) knots 0 0 0 1 1 1
extrude "Extrude42" add sketch "Sketch10" along normal blind 0.25 contours L12 L13 S0 S1 L14 S2 S3 L15 L16 | S4 S5 S6 S7 S8 S9 S10 S11 S12 S13 S14 S15 | S24 S25 S26 S27 S28 S29 S30 S31 S32 S33 S34 S35 | L17 S44 S45 S46 S47 S48 L18 L19 L20 S49 S50 S51 S52 S53 S54 L21 L22 L23 L24 | L25 L26 L27 S55 S56 S57 S58 S59 S60 S61 L28 L29 L30 S62 S63 S64 S65 S66 L31 L32 L33 S67 S68 S69 S70 S71 L34 L35 | L36 L37 L38 L39 | L40 L41 S72 S73 L42 S74 S75 L43 L44 | S76 S77 S78 S79 S80 S81 S82 S83 S84 S85 S86 S87 | S96 S97 S98 S99 S100 S101 S102 S103 S104 S105 S106 S107 | S116 S117 S118 S119 S120 S121 S122 S123 S124 S125 S126 S127 | L45 S136 S137 S138 S139 S140 L46 L47 L48 S141 S142 S143 S144 S145 S146 L49 L50 L51 L52 | L53 L54 L55 S147 S148 S149 S150 S151 S152 S153 L56 L57 L58 S154 S155 S156 S157 S158 L59 L60 L61 S159 S160 S161 S162 S163 L62 L63 | L64 L65 S164 L66 L67 L68 L69 L70 L71 L72 L73 L74 | L98 L99 S307 S308 S309 S310 S311 S312 S313 L100 L101 L102 S314 S315 S316 S317 L103 L104 L105 | L109 S323 S324 S325 S326 S327 S328 S329 S330 S331 L110 S332 S333 S334 S335 | L112 S340 S341 S342 S343 S344 S345 S346 S347 S348 S349 S350 S351 S352 S353 S354 S355 L113 S356 S357 S358 S359 S360 S361 S362 S363 S364 S365 S366 S367 S368 S369 S370 | S371 S372 S373 S374 S375 S376 S377 S378 S379 | L114 L115 L116 L117 | L118 S388 S389 S390 S391 S392 L119 L120 L121 S393 S394 S395 S396 S397 S398 L122 L123 L124 L125 | L126 S399 S400 S401 S402 L127 L128 L129 L130 L131 L132 L133 L134 L135 L136 L137 S403 S404 S405 S406 | L138 L139 L140 L141 | L142 L143 L144 L145 | S407 S408 S409 S410 S411 S412 S413 S414 S415 | L146 L147 L148 S424 S425 S426 S427 S428 L149 L150 L151 S429 S430 S431 S432 S433 L152 L153 | L154 S434 S435 S436 S437 L155 L156 L157 L158 L159 L160 L161 L162 L163 L164 L165 S438 S439 S440 S441 | L166 S442 S443 S444 S445 S446 S447 S448 S449 S450 L167 S451 S452 S453 S454 | L169 S459 S460 S461 S462 S463 S464 S465 S466 S467 S468 S469 S470 S471 S472 S473 S474 L170 S475 S476 S477 S478 S479 S480 S481 S482 S483 S484 S485 S486 S487 S488 S489 | L171 S490 S491 S492 S493 L172 L173 L174 L175 L176 L177 L178 L179 L180 L181 L182 S494 S495 S496 S497 | S498 S499 S500 S501 S502 S503 S504 S505 S506 S507 S508 S509 | L183 S518 S519 S520 S521 S522 S523 S524 S525 S526 L184 L185 L186 L187 | L188 S535 S536 S537 S538 S539 S540 S541 S542 S543 L189 S544 S545 S546 S547 | L191 S552 S553 S554 S555 S556 S557 S558 S559 S560 S561 S562 S563 L192 L193 L194 S564 S565 S566 S567 S568
extrude "Extrude41" [suppressed]
